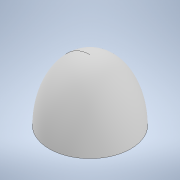
# Autodesk Inventor part: Top Inside
Saved by Autodesk Inventor 2022 (Build 260153000, 153)
## iProperties
Created: 2022-03-08
Part Number: Top Inside
Material: Generic
Document SubType Name: Modeling
Designer: Nathan Griffith
Density: 1 g/cm^3
Appearance: Default
Author: Nathan Griffith
Autodesk Inventor part; units mm, degrees
ref_plane "YZ Plane" through (0, 0, 0) normal (1, 0, 0) x (0, 1, 0)
ref_plane "XZ Plane" through (0, 0, 0) normal (0, 1, 0) x (-1, 0, 0)
ref_plane "XY Plane" through (0, 0, 0) normal (0, 0, 1) x (1, 0, 0)
sketch "Sketch1" plane through (0, 0, 0) normal (0, 0, 1) x (1, 0, 0)
  line L0 (-19.05, 25.4) -> (-38.1, 25.4) construction
  ellipse E0 centre (-19.05, 19.05) end of major axis (-19.05, 50.8) minor radius 19.05 (-19.05, 50.8) -> (-38.1, 19.05) ccw
  line L1 (-19.05, 50.8) -> (-19.05, 19.05)
  line L2 (-19.05, 19.05) -> (-38.1, 19.05)
  point P0 (0, 0)
  constraints: 6 end point, 1 point on line, 1 vertical, 4 other
revolve "Revolution1" add sketch "Sketch1" angle 360 about axis through (-19.05, 50.8, 0) along (0, -1, 0)
shell "Shell1" thickness 6.35 outward yes removed faces 1 at (-23.803, 19.05, -4.2108)
body "Solid1"
